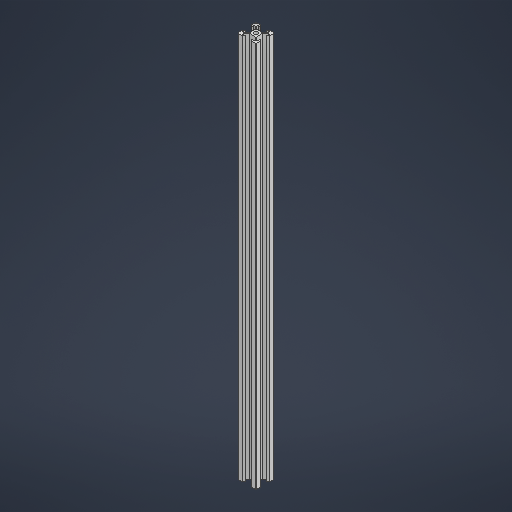
# Autodesk Inventor part: VSLOT20x20x400
Saved by Autodesk Inventor 2026.2 (Build 302298010, 298A)
## iProperties
Created: 2026-04-14
Part Number: VSLOT20x20x400
Material: Generic
Document SubType Name: Modeling
Designer: grego
Density: 1 g/cm^3
Appearance: Default
Author: grego
Autodesk Inventor part; units mm, degrees
ref_plane "YZ Plane" through (0, 0, 0) normal (1, 0, 0) x (0, 1, 0)
ref_plane "XZ Plane" through (0, 0, 0) normal (0, 1, 0) x (-1, 0, 0)
ref_plane "XY Plane" through (0, 0, 0) normal (0, 0, 1) x (1, 0, 0)
sketch "Sketch1" plane through (0, 0, 0) normal (0, 1, 0) x (-1, 0, 0)
  line L0 (3.9, -2.8393) -> (3.9, 2.8393)
  line L1 (2.8393, 3.9) -> (-2.8393, 3.9)
  line L2 (-2.8393, -3.9) -> (2.8393, -3.9)
  line L3 (8.5707, 3.2957) -> (10, 4.725)
  line L4 (8.5707, -3.2957) -> (10, -4.725)
  line L5 (8.4, 3.3664) -> (8.4, 6)
  line L6 (8.4, 6) -> (7.0607, 6)
  line L7 (10, 9) -> (10, 4.725)
  line L8 (10, -4.725) -> (10, -9)
  line L9 (3.9, 2.8393) -> (7.0607, 6)
  line L10 (3.2957, 8.5707) -> (4.725, 10)
  line L11 (3.3664, 8.4) -> (6, 8.4)
  line L12 (6, 8.4) -> (6, 7.0607)
  line L13 (2.8393, 3.9) -> (6, 7.0607)
  line L14 (3.9, 0) -> (8.4, 0)
  line L15 (8.4, -3.3664) -> (8.4, -6)
  line L16 (8.4, -6) -> (7.0607, -6)
  line L17 (3.9, -2.8393) -> (7.0607, -6)
  line L18 (3.2957, -8.5707) -> (4.725, -10)
  line L19 (3.3664, -8.4) -> (6, -8.4)
  line L20 (6, -8.4) -> (6, -7.0607)
  line L21 (2.8393, -3.9) -> (6, -7.0607)
  line L22 (-3.9, -2.8393) -> (-3.9, 2.8393)
  line L23 (-8.5707, 3.2957) -> (-10, 4.725)
  line L24 (-8.5707, -3.2957) -> (-10, -4.725)
  line L25 (-8.4, 3.3664) -> (-8.4, 6)
  line L26 (-8.4, 6) -> (-7.0607, 6)
  line L27 (-10, 9) -> (-10, 4.725)
  line L28 (-10, -4.725) -> (-10, -9)
  line L29 (-3.9, 2.8393) -> (-7.0607, 6)
  line L30 (-3.2957, 8.5707) -> (-4.725, 10)
  line L31 (-3.3664, 8.4) -> (-6, 8.4)
  line L32 (-6, 8.4) -> (-6, 7.0607)
  line L33 (-2.8393, 3.9) -> (-6, 7.0607)
  line L34 (-3.9, -2.8393) -> (-7.0607, -6)
  line L35 (-8.4, -6) -> (-7.0607, -6)
  line L36 (-8.4, -3.3664) -> (-8.4, -6)
  line L37 (-2.8393, -3.9) -> (-6, -7.0607)
  line L38 (-6, -8.4) -> (-6, -7.0607)
  line L39 (-3.3664, -8.4) -> (-6, -8.4)
  line L40 (-3.2957, -8.5707) -> (-4.725, -10)
  line L41 (-9, 10) -> (-4.725, 10)
  line L42 (4.725, 10) -> (9, 10)
  line L43 (9, -10) -> (4.725, -10)
  line L44 (-4.725, -10) -> (-9, -10)
  circle A0 centre (0, 0) radius 2.1
  arc A1 (10, 9) -> (9, 10) centre (9, 9) ccw
  arc A2 (9, -10) -> (10, -9) centre (9, -9) ccw
  arc A3 (-10, -9) -> (-9, -10) centre (-9, -9) ccw
  arc A4 (-9, 10) -> (-10, 9) centre (-9, 9) ccw
  arc A5 (8.4, 3.3664) -> (8.5707, 3.2957) centre (8.5, 3.3664) ccw
  arc A6 (3.2957, 8.5707) -> (3.3664, 8.4) centre (3.3664, 8.5) ccw
  arc A7 (8.5707, -3.2957) -> (8.4, -3.3664) centre (8.5, -3.3664) ccw
  arc A8 (3.3664, -8.4) -> (3.2957, -8.5707) centre (3.3664, -8.5) ccw
  arc A9 (-3.2957, -8.5707) -> (-3.3664, -8.4) centre (-3.3664, -8.5) ccw
  arc A10 (-8.4, -3.3664) -> (-8.5707, -3.2957) centre (-8.5, -3.3664) ccw
  arc A11 (-8.5707, 3.2957) -> (-8.4, 3.3664) centre (-8.5, 3.3664) ccw
  arc A12 (-3.3664, 8.4) -> (-3.2957, 8.5707) centre (-3.3664, 8.5) ccw
  dimension "d11" = 1
  constraints: 90 end point, 24 point on circle, 24 tangent, 13 centre point, 10 equal radius, 7 symmetric about line, 6 perpendicular, 5 parallel, 3 horizontal, 1 midpoint
  measures "d11" radius of A1
extrude "Extrusion1" add sketch "Sketch1" along normal blind 420
body "Solid1"
